IKEA LACK (Autodesk Fusion 360 design; units mm, degrees)
Autodesk Fusion 360 part; units mm, degrees
sketch "Sketch1" plane through (0, 0, 0) normal (0, 0, 1) x (1, 0, 0)
  line L0 (0, 0) -> (550, 0)
  line L1 (550, 0) -> (550, 550)
  line L2 (550, 550) -> (0, 550)
  line L3 (0, 550) -> (0, 0)
  dimension "d1" = 550
  dimension "d2" = 550
  constraint horizontal L0
  constraint vertical L1
  constraint horizontal L2
  constraint vertical L3
  constraint coincident L0.start L3.end
  measures "d1" distance of L0.start L0.end
  measures "d2" distance of L0.start L2.end
extrude "Extrude1" add sketch "Sketch1" along normal blind 50 makes body 1
sketch "Sketch2" plane through (0, 0, 0) normal (0, 0, -1) x (1, 0, 0)
  line L0 (0, 0) -> (0, -550)
  line L1 (0, -550) -> (550, -550)
  line L2 (550, -550) -> (550, 0)
  line L3 (550, 0) -> (0, 0)
  line L4 (2, -2) -> (52.6, -2)
  line L5 (52.6, -2) -> (52.6, -52.6)
  line L6 (52.6, -52.6) -> (2, -52.6)
  line L7 (2, -52.6) -> (2, -2)
  line L8 (497.4, -52.6) -> (497.4, -2)
  line L9 (497.4, -2) -> (548, -2)
  line L10 (548, -2) -> (548, -52.6)
  line L11 (548, -52.6) -> (497.4, -52.6)
  line L12 (2, -548) -> (2, -497.4)
  line L13 (2, -497.4) -> (52.6, -497.4)
  line L14 (52.6, -497.4) -> (52.6, -548)
  line L15 (52.6, -548) -> (2, -548)
  line L16 (497.4, -548) -> (497.4, -497.4)
  line L17 (497.4, -497.4) -> (548, -497.4)
  line L18 (548, -497.4) -> (548, -548)
  line L19 (548, -548) -> (497.4, -548)
  dimension "d5" = 50.6
  dimension "d6" = 50.6
  dimension "d7" = 2
  dimension "d8" = 2
  dimension "d11" = 495.4
  dimension "d12" = -495.4
  constraint horizontal L4
  constraint vertical L5
  constraint horizontal L6
  constraint vertical L7
  measures "d5" distance of L4.start L4.end
  measures "d6" distance of L4.start L6.end
  measures "d7" distance of L0 L7
  measures "d8" distance of L3 L4
extrude "Extrude2" add sketch "Sketch2" along normal blind 400 separate body contours L4 L5 L6 L7 | L8 L9 L10 L11 | L12 L13 L14 L15 | L16 L17 L18 L19 makes body 2 at (497.4, 35.7333, -133.3333) makes body 3 at (497.4, 531.1333, -133.3333) makes body 4 at (18.8667, 2, -133.3333) makes body 5 at (18.8667, 497.4, -133.3333)
equation "d8 = d7"
equation "d11 = d1 - 2 * d7 - d5"
equation "d12 = -d1 + 2 * d7 + d5"
